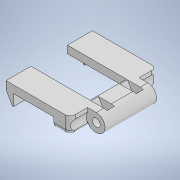
# Autodesk Inventor part: Крепление камеры к корпусу
Saved by Autodesk Inventor 2020 (Build 240168000, 168)
## iProperties
Created: 2021-09-19
Part Number: Крепление камеры к корпусу
Material: Типовые
Document SubType Name: Modeling
Designer: Антон
Density: 1 g/cm^3
Appearance: По умолчанию
Author: Антон
Autodesk Inventor part; units mm, degrees
ref_plane "YZ Plane" through (0, 0, 0) normal (1, 0, 0) x (0, 1, 0)
ref_plane "XZ Plane" through (0, 0, 0) normal (0, 1, 0) x (-1, 0, 0)
sketch "Эскиз1" plane through (0, 0, 0) normal (0, 1, 0) x (-1, 0, 0)
  line L0 (0, 0) -> (23.65, 0)
  line L1 (23.65, 0) -> (23.65, -10)
  line L2 (23.65, -10) -> (0, -10)
  line L3 (0, -10) -> (0, 0)
  line L4 (0, 0) -> (-9, 0)
  line L5 (-9, 0) -> (-9, -17.3)
  line L6 (-9, -17.3) -> (0, -17.3)
  line L7 (0, -17.3) -> (0, 0)
  line L8 (-9, 0) -> (-2, 0)
  line L9 (-2, 0) -> (-2, -7)
  line L10 (-2, -7) -> (-9, -7)
  line L11 (-9, -7) -> (-9, 0)
  point P0 (0, -7)
  point P1 (-9, -7)
  point P2 (-2, 0)
  dimension "d0" = 10
  dimension "d1" = 23.65
  dimension "d2" = 9
  dimension "d3" = 17.3
  dimension "d21" = 7
  dimension "d22" = 7
  constraints: 24 end point, 6 parallel, 3 horizontal, 3 perpendicular
  measures "d0" distance of L0.end L1.end
  measures "d1" distance of L1.end L2.end
  measures "d2" distance of L0.start L4.end
  measures "d3" distance of L4.end L5.end
  measures "d21" distance between parallel lines of L4 L10
  measures "d22" distance of L9.end L10.end
extrude "Выдавливание1" add sketch "Эскиз1" along normal blind 3 contours L0 L1 L2 L3 | L3 L7 L6 L5 L10 L9 L4
sketch "Эскиз2" plane through (0, 0, 0) normal (0, -1, 0) x (1, 0, 0)
  line L0 (-23.65, 0) -> (-20.65, 0)
  line L1 (-20.65, 0) -> (-20.65, -6)
  line L2 (-20.65, -6) -> (-23.65, -6)
  line L3 (-23.65, -6) -> (-23.65, 0)
  point P0 (0, 0)
  dimension "d6" = 6
  dimension "d7" = 3
  constraints: 8 end point, 2 parallel, 1 coincident, 1 horizontal, 1 perpendicular
  measures "d6" distance of L0.end L1.end
  measures "d7" distance of L1.end L2.end
extrude "Выдавливание2" add sketch "Эскиз2" along normal blind 4.5
sketch "Эскиз7" plane through (0, 0, 0) normal (0, -1, 0) x (1, 0, 0)
  line L0 (-23.65, 0) -> (2, 0) projected
  line L1 (2, 0) -> (-4.45, 0)
  line L2 (-4.45, 0) -> (-4.45, -7.9)
  line L3 (-4.45, -7.9) -> (2, -7.9)
  line L4 (2, -7.9) -> (2, 0)
  line L5 (0, -17.3) -> (0, -10) projected
  line L6 (2, -7.9) -> (0, -7.9)
  line L7 (0, -7.9) -> (0, -17.3)
  line L8 (0, -17.3) -> (2, -17.3)
  line L9 (2, -17.3) -> (2, -7.9)
  point P0 (-4.45, 0)
  point P1 (0, -7.9)
  dimension "d26" = 7.9
  dimension "d29" = 6.45
  constraints: 16 end point, 4 parallel, 2 horizontal, 2 perpendicular
  measures "d26" distance of L1.end L2.end
  measures "d29" distance of L2.end L3.end
extrude "Выдавливание5" add sketch "Эскиз7" along normal blind 4
fillet "Сопряжение4" radius 2.225 2 edges at (-4.45, -2, -7.9) (0, -2, -7.9)
fillet "Сопряжение5" radius 2 3 edges at (-1.225, -4, 0) (2, -4, -8.65) (2, -0.5, 0)
chamfer "Фаска1" distance 2.5 distance2 4.5 1 edges at (-23.65, -4.5, -3) measured on face at (-21.65, -4.5, -4)
mirror "Зеркальное отражение1" about plane through (9, 0, -17.3) normal (0, 0, -1)
sketch "Эскиз3" plane through (0, 0, 0) normal (0, 1, 0) x (1, 0, 0)
  line L0 (9, 7) -> (2, 7)
  line L1 (2, 7) -> (2, 27.6)
  line L2 (2, 27.6) -> (9, 27.6)
  line L3 (9, 27.6) -> (9, 7)
  line L4 (2, 7) -> (9, 7) projected
  line L5 (2, 27.6) -> (9, 27.6) projected
  line L6 (9, 7) -> (9, 27.6) projected
  line L7 (2, 2) -> (2, 7) projected
  point P0 (2, 0)
  constraints: 8 end point, 4 collinear, 2 parallel, 1 horizontal, 1 perpendicular
extrude "Выдавливание3" add sketch "Эскиз3" against normal blind 4
fillet "Сопряжение1" radius 3.5 3 edges at (9, -4, -17.3) (2, -4, -17.3) (9, 3, -17.3)
sketch "Эскиз4" plane through (5, 6, -27.6) normal (0, 0, -1) x (1, 0, 0)
  arc A0 (0.5, 3) -> (0.5, 10) centre (0.5, 6.5) ccw projected
hole "Отверстие1" at (5.5, -0.5, -27.6) direction (0, 0, 1) diameter 3.1 end through all
sketch "Эскиз5" plane through (2, 0, -34.6) normal (0, 0, -1) x (-1, 0, 0)
  circle A0 centre (-3.5, -0.5) radius 1.55 projected
  circle A1 centre (-3.5, -0.5) radius 4
  arc A2 (-3.5, 3) -> (-3.5, -4) centre (-3.5, -0.5) ccw projected
  point P0 (2, 0)
  dimension "d37" = 0.5
  constraints: 1 centre point, 1 coincident
  measures "d37" radial gap between concentric circles of A1 A2
extrude "Выдавливание4" cut sketch "Эскиз5" against normal up to surface (7 mm away)
ref_plane "РабПлоскость1" through (-23.65, 3, -17.3) normal (0, 0, 1) x (1, 0, 0)
sketch "Эскиз8" plane through (5.5, 3, -27.6) normal (0, 0, -1) x (-1, 0, 0)
  circle A0 centre (0, -3.5) radius 1.55 projected
  line L0 (1.5588, -0.8) -> (3.1177, -3.5)
  line L1 (3.1177, -3.5) -> (1.5588, -6.2)
  line L2 (1.5588, -6.2) -> (-1.5588, -6.2)
  line L3 (-1.5588, -6.2) -> (-3.1177, -3.5)
  line L4 (-3.1177, -3.5) -> (-1.5588, -0.8)
  line L5 (-1.5588, -0.8) -> (1.5588, -0.8)
  line L6 (3.5, 0) -> (0, 0) projected
  line L7 (-1.5588, -0.8) -> (0.4619, 2.7)
  line L8 (0.4619, 2.7) -> (5.1384, 0)
  line L9 (5.1384, 0) -> (3.1177, -3.5)
  line L10 (3.1177, -3.5) -> (-1.5588, -0.8)
  point P0 (5.5, -3)
  dimension "d41" = 5.4
  constraints: 20 end point, 3 parallel, 1 coincident, 1 perpendicular, 1 point on line, 13 other
  measures "d41" distance between parallel lines of L2 L5
extrude "Выдавливание6" cut sketch "Эскиз8" against normal blind 3 from surface at -3 contours A0 | L5 L7 L8 L9 L0 | L0 L10 L5 | L1 L2 L3 L4 L10
mirror "Зеркальное отражение2" about plane through (-23.65, 3, -17.3) normal (0, 0, 1) of "Выдавливание4", "Выдавливание6"
